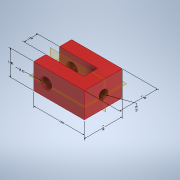
# Autodesk Inventor part: pistonFor-8-in
Saved by Autodesk Inventor 2020.2 (Build 242310000, 310)
## iProperties
Created: 2020-01-13
Part Number: pistonFor-8-in
Material: PET Plastic
Document SubType Name: Modeling
Designer: robst
Density: 1.541 g/cm^3
Appearance: Red
Author: robst
Autodesk Inventor part; units mm, degrees
ref_plane "YZ Plane" through (0, 0, 0) normal (1, 0, 0) x (0, 1, 0)
sketch "Sketch2" plane through (0, 0, 0) normal (0, 0, 1) x (1, 0, 0)
  line L0 (-25.4, -12.7) -> (25.4, -12.7)
  line L1 (25.4, -12.7) -> (25.4, 12.7)
  line L2 (25.4, 12.7) -> (-25.4, 12.7)
  line L3 (-25.4, 12.7) -> (-25.4, -12.7)
  line L4 (-25.4, -12.7) -> (25.4, 12.7) construction
  line L5 (25.4, -12.7) -> (-25.4, 12.7) construction
  point P0 (0, 0)
  dimension "d4" = 50.8
  dimension "d5" = 25.4
  constraints: 12 end point, 2 midpoint, 2 parallel, 1 horizontal, 1 perpendicular
  measures "d4" distance of L0.start L0.end
  measures "d5" distance of L1.end L0.end
extrude "Extrusion2" add sketch "Sketch2" along normal mid plane 38.1
sketch "Sketch3" plane through (-25.4, 12.7, 19.05) normal (0, 1, 0) x (1, 0, 0)
  line L0 (0, 0) -> (0, 38.1) construction
  line L1 (38.1, 19.05) -> (38.1, 25.908)
  line L2 (38.1, 25.908) -> (0, 25.908)
  line L3 (0, 25.908) -> (0, 19.05)
  line L4 (0, 0) -> (0, 25.4) construction
  line L5 (38.1, 19.05) -> (38.1, 12.192)
  line L6 (38.1, 12.192) -> (0, 12.192)
  line L7 (0, 12.192) -> (0, 19.05)
  line L8 (50.8, 0) -> (0, 0) projected
  point P0 (25.4, 19.05)
  dimension "d8" = 38.1
  dimension "d10" = 13.716
  dimension "d34" = 12.192
  constraints: 14 end point, 1 midpoint, 1 parallel
  measures "d8" distance of L2.end L1.end
  measures "d10" distance between parallel lines of L6 L2
  measures "d34" distance between parallel lines of L6 L8
extrude "Extrusion3" cut sketch "Sketch3" against normal through all
sketch "Sketch4" plane through (0, 0, 19.05) normal (0, 0, 1) x (1, 0, 0)
  circle A0 centre (-12.7, 0) radius 5.2705
  line L0 (-25.4, 12.7) -> (-25.4, -12.7) projected
  point P0 (0, 0)
  dimension "d13" = 10.541
  dimension "d14" = 12.7
  constraints: 1 centre point
  measures "d13" diameter of A0
  measures "d14" distance from line of L0 A0.centre
extrude "Extrusion4" cut sketch "Sketch4" against normal through all
sketch "Sketch5" plane through (25.4, -12.7, 19.05) normal (1, 0, 0) x (0, 0, -1)
  circle A0 centre (19.05, 12.7) radius 4.2164
  dimension "d27" = 8.4328
  constraints: 1 centre point, 1 coincident
  measures "d27" diameter of A0
extrude "Extrusion5" cut sketch "Sketch5" against normal blind 12.7
body "Solid2"
